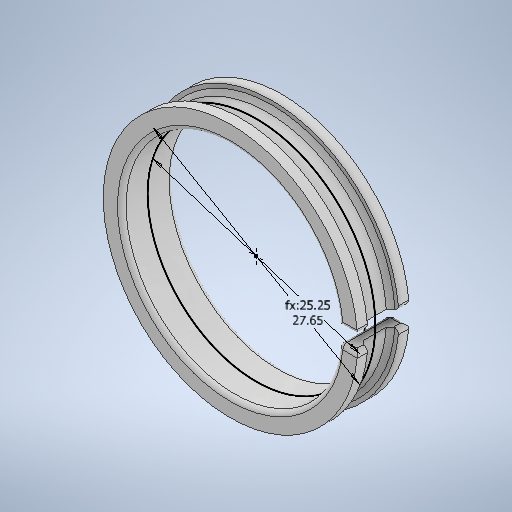
# Autodesk Inventor part: maxtubingBoreWireProtectInsert
Saved by Autodesk Inventor 2025 (Build 290162000, 162)
## iProperties
Created: 2025-03-16
Part Number: maxtubingBoreWireProtectInsert
Material: Generic
Document SubType Name: Modeling
Designer: john
Density: 1 g/cm^3
Appearance: Default
Author: john
Autodesk Inventor part; units mm, degrees
ref_plane "YZ Plane" through (0, 0, 0) normal (1, 0, 0) x (0, 1, 0)
ref_plane "XZ Plane" through (0, 0, 0) normal (0, 1, 0) x (-1, 0, 0)
ref_plane "XY Plane" through (0, 0, 0) normal (0, 0, 1) x (1, 0, 0)
sketch "Sketch1" plane through (0, 0, 0) normal (0, 0, 1) x (1, 0, 0)
  circle A0 centre (0, 0) radius 13.825
  circle A1 centre (0, 0) radius 12.625
  dimension "d0" = 27.65
  dimension "d1" = 25.25
  constraints: 3 coincident, 2 centre point
  measures "d0" diameter of A0
  measures "d1" diameter of A1
extrude "Extrusion1" add sketch "Sketch1" along normal blind 1.8
sketch "Sketch2" plane through (0, 0, 1.8) normal (0, 0, 1) x (1, 0, 0)
  circle A0 centre (0, 0) radius 12.625
  circle A1 centre (0, 0) radius 14.775
  dimension "d5" = 29.55
  dimension "d16" = 25.25
  constraints: 3 coincident, 2 centre point
  measures "d5" diameter of A1
  measures "d16" diameter of A0
extrude "Extrusion2" add sketch "Sketch2" along normal blind 1.2
sketch "Sketch3" plane through (0, 0, 0) normal (0, 0, 1) x (1, 0, 0)
  line L0 (11.2898, 0.9) -> (17.9351, 0.9)
  line L1 (17.9351, 0.9) -> (17.9351, -0.9)
  line L2 (17.9351, -0.9) -> (11.2898, -0.9)
  line L3 (11.2898, -0.9) -> (11.2898, 0.9)
  point P0 (0, 0)
  dimension "d13" = 1.8
  dimension "d14" = 6.6453
  dimension "d15" = 0.9
  constraints: 8 end point, 2 parallel, 1 horizontal, 1 perpendicular
  measures "d13" distance between parallel lines of L2 L0
  measures "d14" distance of L0.start L0.end
  measures "d15" distance from line of point (0, 0) L0
extrude "Extrusion3" cut sketch "Sketch3" along normal blind 6
chamfer "Chamfer1" distance 0.5 angle 45 1 edges at (-13.825, 0, 1.8)
mirror "Mirror2" about plane through (0, 0, 0) normal (0, 0, 1) of "Extrusion1", "Extrusion2", "Extrusion3", "Chamfer1"
fillet "Fillet1" radius 0.5 11 edges at (-12.625, 0, 3) (-12.625, 0, -3) (12.5929, -0.9, 0) (13.6702, -0.9, 3) (13.6702, -0.9, -3) (13.6702, 0.9, 3) (13.6702, 0.9, -3) (14.7476, 0.9, 2.4) (14.7476, 0.9, -2.4) (14.7476, -0.9, -2.4) (14.7476, -0.9, 2.4)
equation "\"d16\" = d1"
equation "\"d15\" = 0.5 * d13"
body "Solid1"
